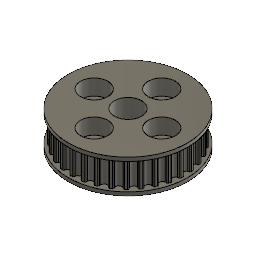
grt_cardan_joint_pulley_33T_20190328 (Autodesk Fusion 360 design; units mm, degrees)
Autodesk Fusion 360 part; units mm, degrees
(part 1 of 2)
sketch "Skizze1" plane through (0, 0, 0) normal (0, 1, 0) x (1, 0, 0)
  line L0 (0, 16.3863) -> (0, 0) construction
  arc A0 (-0.7739, 14.4848) -> (0, 13.9863) centre (0, 14.8363) ccw
  arc A1 (-0.8908, 14.8724) -> (-0.7739, 14.4848) centre (0.61, 15.1135) ccw
  arc A2 (-0.8908, 14.8724) -> (-1.1567, 15.082) centre (-1.1376, 14.8328) ccw
  arc A3 (0, 16.0053) -> (-1.5214, 15.9329) centre (0, 0) ccw construction
  arc A4 (-1.1567, 15.082) -> (-1.4378, 15.0578) centre (0, 0) ccw
  arc A5 (0, 16.3863) -> (-1.5576, 16.3121) centre (0, 0) ccw construction
  line L1 (0, 0) -> (-1.5576, 16.3121) construction
  line L2 (-1.4378, 15.0578) -> (0, 0)
  line L3 (0, 13.9863) -> (0, 0)
  dimension "d2" = 1.14
  dimension "d4" = 0.85
  dimension "d5" = 1.52
  dimension "d6" = 0.25
  dimension "d7" = 0.61
  dimension "d8" = 0.381
  dimension "d12" = 1.26
  dimension "d19" = 5.455
  dimension "d24" = 2.4
  dimension "d131" = 13.9863
  dimension "d133" = 14.6489
  measures "d4" radius of A0
  measures "d5" radius of A1
  measures "d6" radius of A2
  measures "d7" distance of L0
  measures "d19" angle of L0 L1
  measures "d131" distance of L0.end
  measures "d133" distance of L0.end
extrude "Extrusion1" add sketch "Skizze1" along normal blind 7 makes body 1
mirror "Spiegeln1" about plane through (0, 0, -13.9863) normal (1, 0, 0) of bodies 1 makes body 2
combine "Kombinieren1" operation add target body 1 tool bodies 2
pattern_circular "C-Anordnung1" count 33 over 360 about axis through (0, 1.75, 0) along (0, 1, 0) of bodies 1 makes body 3 at (-0.9586, 2.3333, -10.0386) makes body 4 at (-4.2787, 0, -8.8212) makes body 5 at (-5.8708, 0, -7.852) makes body 6 at (-7.2507, 0, -6.5991) makes body 7 at (-8.3685, 0, -5.1076) makes body 8 at (-9.1839, 0, -3.4316) makes body 9 at (-9.6674, 0, -1.6315) makes body 10 at (-9.8014, 0, 0.2276) makes body 11 at (-9.5812, 0, 2.0784) makes body 12 at (-9.0148, 0, 3.8541) makes body 13 at (-8.1225, 0, 5.4905) makes body 14 at (-6.9366, 0, 6.9285) makes body 15 at (-5.5, 0, 8.116) makes body 16 at (-3.8647, 0, 9.0102) makes body 17 at (-2.0896, 0, 9.5788) makes body 18 at (-0.2391, 0, 9.8012) makes body 19 at (1.6201, 0, 9.6693) makes body 20 at (3.4208, 0, 9.1879) makes body 21 at (5.0978, 0, 8.3745) makes body 22 at (6.5906, 0, 7.2584) makes body 23 at (7.8451, 0, 5.88) makes body 24 at (8.8161, 0, 4.289) makes body 25 at (9.4685, 0, 2.543) makes body 26 at (9.7787, 0, 0.7051) makes body 27 at (9.7354, 0, -1.1582) makes body 28 at (9.3403, 0, -2.9797) makes body 29 at (8.6076, 0, -4.6936) makes body 30 at (7.5638, 0, -6.2377) makes body 31 at (6.2466, 0, -7.5565) makes body 32 at (4.7036, 0, -8.6021) makes body 33 at (2.9907, 0, -9.3368) makes body 34 at (0.9586, 2.3333, -10.0386)
combine "Kombinieren2" operation add target body 1 tool bodies 21 20 19 3 18 17 8 15 7 12 9 11 10 16 6 5 14 4 13 31 27 22 23 29 25 24 26 28 30 33 32
sketch "Skizze2" plane through (0, 7, 0) normal (0, 1, 0) x (-1, 0, 0)
  arc A0 (-1.4378, -15.0578) -> (-1.1567, -15.082) centre (0, 0) ccw
  arc A1 (-1.1567, -15.082) -> (-0.8908, -14.8724) centre (-1.1376, -14.8328) ccw
  arc A2 (-0.7739, -14.4848) -> (-0.8908, -14.8724) centre (0.61, -15.1135) ccw
  arc A3 (0.7739, -14.4848) -> (-0.7739, -14.4848) centre (0, -14.8363) ccw
  arc A4 (0.8908, -14.8724) -> (0.7739, -14.4848) centre (-0.61, -15.1135) ccw
  arc A5 (0.8908, -14.8724) -> (1.1567, -15.082) centre (1.1376, -14.8328) ccw
  arc A6 (1.1567, -15.082) -> (1.7185, -15.0284) centre (0, 0) ccw
  arc A7 (1.7185, -15.0284) -> (1.94, -14.7722) centre (1.6901, -14.78) ccw
  arc A8 (1.9814, -14.3695) -> (1.94, -14.7722) centre (3.4592, -14.7249) ccw
  arc A9 (3.5012, -14.0765) -> (1.9814, -14.3695) centre (2.8078, -14.5682) ccw
  arc A10 (3.6893, -14.4351) -> (3.5012, -14.0765) centre (2.2613, -14.9558) ccw
  arc A11 (3.6893, -14.4351) -> (3.9901, -14.5906) centre (3.9242, -14.3494) ccw
  arc A12 (3.9901, -14.5906) -> (4.5316, -14.4316) centre (0, 0) ccw
  arc A13 (4.5316, -14.4316) -> (4.7006, -14.1381) centre (4.4567, -14.1931) ccw
  arc A14 (4.665, -13.7348) -> (4.7006, -14.1381) centre (6.1834, -13.8041) ccw
  arc A15 (6.1019, -13.1596) -> (4.665, -13.7348) centre (5.5141, -13.7736) ccw
  arc A16 (6.3545, -13.476) -> (6.1019, -13.1596) centre (5.0508, -14.2576) ccw
  arc A17 (6.3545, -13.476) -> (6.6793, -13.5718) centre (6.5689, -13.3475) ccw
  arc A18 (6.6793, -13.5718) -> (7.1809, -13.3132) centre (0, 0) ccw
  arc A19 (7.1809, -13.3132) -> (7.2913, -12.9931) centre (7.0622, -13.0932) ccw
  arc A20 (7.18, -12.6037) -> (7.2913, -12.9931) centre (8.6841, -12.3845) ccw
  arc A21 (8.4821, -11.767) -> (7.18, -12.6037) centre (8.0211, -12.4811) ccw
  arc A22 (8.79, -12.0299) -> (8.4821, -11.767) centre (7.6578, -13.044) ccw
  arc A23 (8.79, -12.0299) -> (9.1271, -12.0625) centre (8.9762, -11.8631) ccw
  arc A24 (9.1271, -12.0625) -> (9.5706, -11.7136) centre (0, 0) ccw
  arc A25 (9.5706, -11.7136) -> (9.6185, -11.3784) centre (9.4125, -11.52) ccw
  arc A26 (9.4355, -11.0172) -> (9.6185, -11.3784) centre (10.871, -10.5172) ccw
  arc A27 (10.5557, -9.9491) -> (9.4355, -11.0172) centre (10.2382, -10.7376) ccw
  arc A28 (10.9078, -10.149) -> (10.5557, -9.9491) centre (9.988, -11.3591) ccw
  arc A29 (10.9078, -10.149) -> (11.245, -10.1172) centre (11.0591, -9.95) ccw
  arc A30 (11.245, -10.1172) -> (11.6145, -9.6907) centre (0, 0) ccw
  arc A31 (11.6145, -9.6907) -> (11.598, -9.3524) centre (11.4226, -9.5305) ccw
  arc A32 (11.35, -9.0324) -> (11.598, -9.3524) centre (12.6649, -8.2698) ccw
  arc A33 (12.2478, -7.7716) -> (11.35, -9.0324) centre (12.0853, -8.6059) ccw
  arc A34 (12.6314, -7.9013) -> (12.2478, -7.7716) centre (11.9572, -9.2636) ccw
  arc A35 (12.6314, -7.9013) -> (12.9564, -7.8062) centre (12.7423, -7.6772) ccw
  arc A36 (12.9564, -7.8062) -> (13.2386, -7.3175) centre (0, 0) ccw
  arc A37 (13.2386, -7.3175) -> (13.1584, -6.9885) centre (13.0198, -7.1966) ccw
  arc A38 (12.8543, -6.7211) -> (13.1584, -6.9885) centre (14.0011, -5.7235) ccw
  arc A39 (13.4973, -5.3132) -> (12.8543, -6.7211) centre (13.4956, -6.1632) ccw
  arc A40 (13.8985, -5.368) -> (13.4973, -5.3132) centre (13.4943, -6.8332) ccw
  arc A41 (13.8985, -5.368) -> (14.1996, -5.2131) centre (13.9649, -5.127) ccw
  arc A42 (14.1996, -5.2131) -> (14.3842, -4.6798) centre (0, 0) ccw
  arc A43 (14.3842, -4.6798) -> (14.2432, -4.372) centre (14.1465, -4.6025) ccw
  arc A44 (13.894, -4.167) -> (14.2432, -4.372) centre (14.8313, -2.9703) ccw
  arc A45 (14.2589, -2.6628) -> (13.894, -4.167) centre (14.4181, -3.4978) ccw
  arc A46 (14.6632, -2.6407) -> (14.2589, -2.6628) centre (14.5436, -4.1559) ccw
  arc A47 (14.6632, -2.6407) -> (14.9296, -2.4316) centre (14.6829, -2.3914) ccw
  arc A48 (14.9296, -2.4316) -> (15.0099, -1.873) centre (0, 0) ccw
  arc A49 (15.0099, -1.873) -> (14.8132, -1.5974) centre (14.7618, -1.8421) ccw
  arc A50 (14.4315, -1.4622) -> (14.8132, -1.5974) centre (15.1254, -0.1098) ccw
  arc A51 (14.5052, 0.0838) -> (14.4315, -1.4622) centre (14.8195, -0.7059) ccw
  arc A52 (14.898, 0.1821) -> (14.5052, 0.0838) centre (15.0673, -1.3284) ccw
  arc A53 (14.898, 0.1821) -> (15.12, 0.4378) centre (14.8701, 0.4305) ccw
  arc A54 (15.12, 0.4378) -> (15.0932, 1.0015) centre (0, 0) ccw
  arc A55 (15.0932, 1.0015) -> (14.8478, 1.2349) centre (14.8437, 0.9849) ccw
  arc A56 (14.4475, 1.2954) -> (14.8478, 1.2349) centre (14.8728, 2.7547) ccw
  arc A57 (14.2272, 2.8274) -> (14.4475, 1.2954) centre (14.6853, 2.1114) ccw
  arc A58 (14.5943, 2.9983) -> (14.2272, 2.8274) centre (15.0464, 1.5471) ccw
  arc A59 (14.5943, 2.9983) -> (14.7639, 3.2913) centre (14.5199, 3.2369) ccw
  arc A60 (14.7639, 3.2913) -> (14.6309, 3.8398) centre (0, 0) ccw
  arc A61 (14.6309, 3.8398) -> (14.3458, 4.0225) centre (14.3891, 3.7763) ccw
  arc A62 (13.9412, 4.0062) -> (14.3458, 4.0225) centre (14.0827, 5.5196) ccw
  arc A63 (13.435, 5.4688) -> (13.9412, 4.0062) centre (14.0204, 4.8525) ccw
  arc A64 (13.7631, 5.7061) -> (13.435, 5.4688) centre (14.4818, 4.3667) ccw
  arc A65 (13.7631, 5.7061) -> (13.8742, 6.026) centre (13.6449, 5.9264) ccw
  arc A66 (13.8742, 6.026) -> (13.6398, 6.5393) centre (0, 0) ccw
  arc A67 (13.6398, 6.5393) -> (13.3253, 6.6648) centre (13.4144, 6.4312) ccw
  arc A68 (12.9311, 6.5722) -> (13.3253, 6.6648) centre (12.7836, 8.085) ccw
  arc A69 (12.1572, 7.9126) -> (12.9311, 6.5722) centre (12.8486, 7.4182) ccw
  arc A70 (12.4345, 8.2076) -> (12.1572, 7.9126) centre (13.3936, 7.0285) ccw
  arc A71 (12.4345, 8.2076) -> (12.4831, 8.5428) centre (12.2768, 8.4016) ccw
  arc A72 (12.4831, 8.5428) -> (12.1557, 9.0024) centre (0, 0) ccw
  arc A73 (12.1557, 9.0024) -> (11.8232, 9.0662) centre (11.9548, 8.8537) ccw
  arc A74 (11.4536, 8.9006) -> (11.8232, 9.0662) centre (11.0225, 10.3582) ccw
  arc A75 (10.4401, 10.0704) -> (11.4536, 8.9006) centre (11.2126, 9.7157) ccw
  arc A76 (10.6565, 10.4126) -> (10.4401, 10.0704) centre (11.8215, 9.4362) ccw
  arc A77 (10.6565, 10.4126) -> (10.6408, 10.7508) centre (10.4649, 10.5731) ccw
  arc A78 (10.6408, 10.7508) -> (10.2323, 11.1403) centre (0, 0) ccw
  arc A79 (10.2323, 11.1403) -> (9.8937, 11.1399) centre (10.0632, 10.9561) ccw
  arc A80 (9.5622, 10.9074) -> (9.8937, 11.1399) centre (8.863, 12.2571) ccw
  arc A81 (8.3456, 11.8642) -> (9.5622, 10.9074) centre (9.1712, 11.6622) ccw
  arc A82 (8.4933, 12.2412) -> (8.3456, 11.8642) centre (9.822, 11.5029) ccw
  arc A83 (8.4933, 12.2412) -> (8.4139, 12.5703) centre (8.2748, 12.3626) ccw
  arc A84 (8.4139, 12.5703) -> (7.9391, 12.8754) centre (0, 0) ccw
  arc A85 (7.9391, 12.8754) -> (7.6067, 12.811) centre (7.8079, 12.6626) ccw
  arc A86 (7.3252, 12.52) -> (7.6067, 12.811) centre (6.3832, 13.7129) ccw
  arc A87 (5.9494, 13.2292) -> (7.3252, 12.52) centre (6.7984, 13.1871) ccw
  arc A88 (6.0232, 13.6273) -> (5.9494, 13.2292) centre (7.4676, 13.1539) ccw
  arc A89 (6.0232, 13.6273) -> (5.8829, 13.9355) centre (5.7856, 13.7052) ccw
  arc A90 (5.8829, 13.9355) -> (5.359, 14.1452) centre (0, 0) ccw
  arc A91 (5.359, 14.1452) -> (5.0447, 14.019) centre (5.2704, 13.9114) ccw
  arc A92 (4.8234, 13.68) -> (5.0447, 14.019) centre (3.6727, 14.6731) ccw
  arc A93 (3.3383, 14.1161) -> (4.8234, 13.68) centre (4.1799, 14.2354) ccw
  arc A94 (3.3354, 14.5209) -> (3.3383, 14.1161) centre (4.8432, 14.3294) ccw
  arc A95 (3.3354, 14.5209) -> (3.1392, 14.797) centre (3.0874, 14.5524) ccw
  arc A96 (3.1392, 14.797) -> (2.5851, 14.9038) centre (0, 0) ccw
  arc A97 (2.5851, 14.9038) -> (2.3004, 14.7204) centre (2.5424, 14.6575) ccw
  arc A98 (2.1472, 14.3456) -> (2.3004, 14.7204) centre (0.8294, 15.103) ccw
  arc A99 (0.6065, 14.4927) -> (2.1472, 14.3456) centre (1.4103, 14.7692) ccw
  arc A100 (0.527, 14.8898) -> (0.6065, 14.4927) centre (2.0439, 14.987) ccw
  arc A101 (0.527, 14.8898) -> (0.2822, 15.1237) centre (0.2775, 14.8738) ccw
  arc A102 (0.2822, 15.1237) -> (-0.2822, 15.1237) centre (0, 0) ccw
  arc A103 (-0.2822, 15.1237) -> (-0.527, 14.8898) centre (-0.2775, 14.8738) ccw
  arc A104 (-0.6065, 14.4927) -> (-0.527, 14.8898) centre (-2.0439, 14.987) ccw
  arc A105 (-2.1472, 14.3456) -> (-0.6065, 14.4927) centre (-1.4103, 14.7692) ccw
  arc A106 (-2.3004, 14.7204) -> (-2.1472, 14.3456) centre (-0.8294, 15.103) ccw
  arc A107 (-2.3004, 14.7204) -> (-2.5851, 14.9038) centre (-2.5424, 14.6575) ccw
  arc A108 (-2.5851, 14.9038) -> (-3.1392, 14.797) centre (0, 0) ccw
  arc A109 (-3.1392, 14.797) -> (-3.3354, 14.5209) centre (-3.0874, 14.5524) ccw
  arc A110 (-3.3383, 14.1161) -> (-3.3354, 14.5209) centre (-4.8432, 14.3294) ccw
  arc A111 (-4.8234, 13.68) -> (-3.3383, 14.1161) centre (-4.1799, 14.2354) ccw
  arc A112 (-5.0447, 14.019) -> (-4.8234, 13.68) centre (-3.6727, 14.6731) ccw
  arc A113 (-5.0447, 14.019) -> (-5.359, 14.1452) centre (-5.2704, 13.9114) ccw
  arc A114 (-5.359, 14.1452) -> (-5.8829, 13.9355) centre (0, 0) ccw
  arc A115 (-5.8829, 13.9355) -> (-6.0232, 13.6273) centre (-5.7856, 13.7052) ccw
  arc A116 (-5.9494, 13.2292) -> (-6.0232, 13.6273) centre (-7.4676, 13.1539) ccw
  arc A117 (-7.3252, 12.52) -> (-5.9494, 13.2292) centre (-6.7984, 13.1871) ccw
  arc A118 (-7.6067, 12.811) -> (-7.3252, 12.52) centre (-6.3832, 13.7129) ccw
  arc A119 (-7.6067, 12.811) -> (-7.9391, 12.8754) centre (-7.8079, 12.6626) ccw
  arc A120 (-7.9391, 12.8754) -> (-8.4139, 12.5703) centre (0, 0) ccw
  arc A121 (-8.4139, 12.5703) -> (-8.4933, 12.2412) centre (-8.2748, 12.3626) ccw
  arc A122 (-8.3456, 11.8642) -> (-8.4933, 12.2412) centre (-9.822, 11.5029) ccw
  arc A123 (-9.5622, 10.9074) -> (-8.3456, 11.8642) centre (-9.1712, 11.6622) ccw
  arc A124 (-9.8937, 11.1399) -> (-9.5622, 10.9074) centre (-8.863, 12.2571) ccw
  arc A125 (-9.8937, 11.1399) -> (-10.2323, 11.1403) centre (-10.0632, 10.9561) ccw
  arc A126 (-10.2323, 11.1403) -> (-10.6408, 10.7508) centre (0, 0) ccw
  arc A127 (-10.6408, 10.7508) -> (-10.6565, 10.4126) centre (-10.4649, 10.5731) ccw
  arc A128 (-10.4401, 10.0704) -> (-10.6565, 10.4126) centre (-11.8215, 9.4362) ccw
  arc A129 (-11.4536, 8.9006) -> (-10.4401, 10.0704) centre (-11.2126, 9.7157) ccw
  arc A130 (-11.8232, 9.0662) -> (-11.4536, 8.9006) centre (-11.0225, 10.3582) ccw
  arc A131 (-11.8232, 9.0662) -> (-12.1557, 9.0024) centre (-11.9548, 8.8537) ccw
  arc A132 (-12.1557, 9.0024) -> (-12.4831, 8.5428) centre (0, 0) ccw
  arc A133 (-12.4831, 8.5428) -> (-12.4345, 8.2076) centre (-12.2768, 8.4016) ccw
  arc A134 (-12.1572, 7.9126) -> (-12.4345, 8.2076) centre (-13.3936, 7.0285) ccw
  arc A135 (-12.9311, 6.5722) -> (-12.1572, 7.9126) centre (-12.8486, 7.4182) ccw
  arc A136 (-13.3253, 6.6648) -> (-12.9311, 6.5722) centre (-12.7836, 8.085) ccw
  arc A137 (-13.3253, 6.6648) -> (-13.6398, 6.5393) centre (-13.4144, 6.4312) ccw
  arc A138 (-13.6398, 6.5393) -> (-13.8742, 6.026) centre (0, 0) ccw
  arc A139 (-13.8742, 6.026) -> (-13.7631, 5.7061) centre (-13.6449, 5.9264) ccw
  arc A140 (-13.435, 5.4688) -> (-13.7631, 5.7061) centre (-14.4818, 4.3667) ccw
  arc A141 (-13.9412, 4.0062) -> (-13.435, 5.4688) centre (-14.0204, 4.8525) ccw
  arc A142 (-14.3458, 4.0225) -> (-13.9412, 4.0062) centre (-14.0827, 5.5196) ccw
  arc A143 (-14.3458, 4.0225) -> (-14.6309, 3.8398) centre (-14.3891, 3.7763) ccw
  arc A144 (-14.6309, 3.8398) -> (-14.7639, 3.2913) centre (0, 0) ccw
  arc A145 (-14.7639, 3.2913) -> (-14.5943, 2.9983) centre (-14.5199, 3.2369) ccw
  arc A146 (-14.2272, 2.8274) -> (-14.5943, 2.9983) centre (-15.0464, 1.5471) ccw
  arc A147 (-14.4475, 1.2954) -> (-14.2272, 2.8274) centre (-14.6853, 2.1114) ccw
  arc A148 (-14.8478, 1.2349) -> (-14.4475, 1.2954) centre (-14.8728, 2.7547) ccw
  arc A149 (-14.8478, 1.2349) -> (-15.0932, 1.0015) centre (-14.8437, 0.9849) ccw
  arc A150 (-15.0932, 1.0015) -> (-15.12, 0.4378) centre (0, 0) ccw
  arc A151 (-15.12, 0.4378) -> (-14.898, 0.1821) centre (-14.8701, 0.4305) ccw
  arc A152 (-14.5052, 0.0838) -> (-14.898, 0.1821) centre (-15.0673, -1.3284) ccw
  arc A153 (-14.4315, -1.4622) -> (-14.5052, 0.0838) centre (-14.8195, -0.7059) ccw
  arc A154 (-14.8132, -1.5974) -> (-14.4315, -1.4622) centre (-15.1254, -0.1098) ccw
  arc A155 (-14.8132, -1.5974) -> (-15.0099, -1.873) centre (-14.7618, -1.8421) ccw
  arc A156 (-15.0099, -1.873) -> (-14.9296, -2.4316) centre (0, 0) ccw
  arc A157 (-14.9296, -2.4316) -> (-14.6632, -2.6407) centre (-14.6829, -2.3914) ccw
  arc A158 (-14.2589, -2.6628) -> (-14.6632, -2.6407) centre (-14.5436, -4.1559) ccw
  arc A159 (-13.894, -4.167) -> (-14.2589, -2.6628) centre (-14.4181, -3.4978) ccw
  arc A160 (-14.2432, -4.372) -> (-13.894, -4.167) centre (-14.8313, -2.9703) ccw
  arc A161 (-14.2432, -4.372) -> (-14.3842, -4.6798) centre (-14.1465, -4.6025) ccw
  arc A162 (-14.3842, -4.6798) -> (-14.1996, -5.2131) centre (0, 0) ccw
  arc A163 (-14.1996, -5.2131) -> (-13.8985, -5.368) centre (-13.9649, -5.127) ccw
  arc A164 (-13.4973, -5.3132) -> (-13.8985, -5.368) centre (-13.4943, -6.8332) ccw
  arc A165 (-12.8543, -6.7211) -> (-13.4973, -5.3132) centre (-13.4956, -6.1632) ccw
  arc A166 (-13.1584, -6.9885) -> (-12.8543, -6.7211) centre (-14.0011, -5.7235) ccw
  arc A167 (-13.1584, -6.9885) -> (-13.2386, -7.3175) centre (-13.0198, -7.1966) ccw
  arc A168 (-13.2386, -7.3175) -> (-12.9564, -7.8062) centre (0, 0) ccw
  arc A169 (-12.9564, -7.8062) -> (-12.6314, -7.9013) centre (-12.7423, -7.6772) ccw
  arc A170 (-12.2478, -7.7716) -> (-12.6314, -7.9013) centre (-11.9572, -9.2636) ccw
  arc A171 (-11.35, -9.0324) -> (-12.2478, -7.7716) centre (-12.0853, -8.6059) ccw
  arc A172 (-11.598, -9.3524) -> (-11.35, -9.0324) centre (-12.6649, -8.2698) ccw
  arc A173 (-11.598, -9.3524) -> (-11.6145, -9.6907) centre (-11.4226, -9.5305) ccw
  arc A174 (-11.6145, -9.6907) -> (-11.245, -10.1172) centre (0, 0) ccw
  arc A175 (-11.245, -10.1172) -> (-10.9078, -10.149) centre (-11.0591, -9.95) ccw
  arc A176 (-10.5557, -9.9491) -> (-10.9078, -10.149) centre (-9.988, -11.3591) ccw
  arc A177 (-9.4355, -11.0172) -> (-10.5557, -9.9491) centre (-10.2382, -10.7376) ccw
  arc A178 (-9.6185, -11.3784) -> (-9.4355, -11.0172) centre (-10.871, -10.5172) ccw
  arc A179 (-9.6185, -11.3784) -> (-9.5706, -11.7136) centre (-9.4125, -11.52) ccw
  circle A180 centre (0, 0) radius 16.3753
  arc A181 (-9.5706, -11.7136) -> (-9.1271, -12.0625) centre (0, 0) ccw
  arc A182 (-9.1271, -12.0625) -> (-8.79, -12.0299) centre (-8.9762, -11.8631) ccw
  arc A183 (-8.4821, -11.767) -> (-8.79, -12.0299) centre (-7.6578, -13.044) ccw
  arc A184 (-7.18, -12.6037) -> (-8.4821, -11.767) centre (-8.0211, -12.4811) ccw
  arc A185 (-7.2913, -12.9931) -> (-7.18, -12.6037) centre (-8.6841, -12.3845) ccw
  arc A186 (-7.2913, -12.9931) -> (-7.1809, -13.3132) centre (-7.0622, -13.0932) ccw
  arc A187 (-7.1809, -13.3132) -> (-6.6793, -13.5718) centre (0, 0) ccw
  arc A188 (-6.6793, -13.5718) -> (-6.3545, -13.476) centre (-6.5689, -13.3475) ccw
  arc A189 (-6.1019, -13.1596) -> (-6.3545, -13.476) centre (-5.0508, -14.2576) ccw
  arc A190 (-4.665, -13.7348) -> (-6.1019, -13.1596) centre (-5.5141, -13.7736) ccw
  arc A191 (-4.7006, -14.1381) -> (-4.665, -13.7348) centre (-6.1834, -13.8041) ccw
  arc A192 (-4.7006, -14.1381) -> (-4.5316, -14.4316) centre (-4.4567, -14.1931) ccw
  arc A193 (-4.5316, -14.4316) -> (-4.2616, -14.5136) centre (0, 0) ccw
  line L0 (-4.2616, -14.5136) -> (0, 0)
  line L1 (0, 0) -> (-1.4378, -15.0578)
  dimension "d30" = 32.7507
  measures "d30" diameter of A180
extrude "Extrusion2" add sketch "Skizze2" along normal blind 1 contours A0 A1 A2 A3 A4 A5 A6 A7 A8 A9 A10 A11 A12 A13 A14 A15 A16 A17 A18 A19 A20 A21 A22 A23 A24 A25 A26 A27 A28 A29 A30 A31 A32 A33 A34 A35 A36 A37 A38 A39 A40 A41 A42 A43 A44 A45 A46 A47 A48 A49 A50 A51 A52 A53 A54 A55 A56 A57 A58 A59 A60 A61 A62 A63 A64 A65 A66 A67 A68 A69 A70 A71 A72 A73 A74 A75 A76 A77 A78 A79 A80 A81 A82 A83 A84 A85 A86 A87 A88 A89 A90 A91 A92 A93 A94 A95 A96 A97 A98 A99 A100 A101 A102 A103 A104 A105 A106 A107 A108 A109 A110 A111 A112 A113 A114 A115 A116 A117 A118 A119 A120 A121 A122 A123 A124 A125 A126 A127 A128 A129 A130 A131 A132 A133 A134 A135 A136 A137 A138 A139 A140 A141 A142 A143 A144 A145 A146 A147 A148 A149 A150 A151 A152 A153 A154 A155 A156 A157 A158 A159 A160 A161 A162 A163 A164 A165 A166 A167 A168 A169 A170 A171 A172 A173 A174 A175 A176 A177 A178 A179 A181 A182 A183 A184 A185 A186 A187 A188 A189 A190 A191 A192 A193 L0 L1 | A180 bodies 1 34
sketch "Skizze3" plane through (0, 0, 0) normal (0, -1, 0) x (1, 0, 0)
  arc A0 (9.5706, -11.7136) -> (9.6185, -11.3784) centre (9.4125, -11.52) ccw
  arc A1 (9.4355, -11.0172) -> (9.6185, -11.3784) centre (10.871, -10.5172) ccw
  arc A2 (10.5557, -9.9491) -> (9.4355, -11.0172) centre (10.2382, -10.7376) ccw
  arc A3 (10.9078, -10.149) -> (10.5557, -9.9491) centre (9.988, -11.3591) ccw
  arc A4 (10.9078, -10.149) -> (11.245, -10.1172) centre (11.0591, -9.95) ccw
  arc A5 (11.245, -10.1172) -> (11.6145, -9.6907) centre (0, 0) ccw
  arc A6 (11.6145, -9.6907) -> (11.598, -9.3524) centre (11.4226, -9.5305) ccw
  arc A7 (11.35, -9.0324) -> (11.598, -9.3524) centre (12.6649, -8.2698) ccw
  arc A8 (12.2478, -7.7716) -> (11.35, -9.0324) centre (12.0853, -8.6059) ccw
  arc A9 (12.6314, -7.9013) -> (12.2478, -7.7716) centre (11.9572, -9.2636) ccw
  arc A10 (12.6314, -7.9013) -> (12.9564, -7.8062) centre (12.7423, -7.6772) ccw
  arc A11 (12.9564, -7.8062) -> (13.2386, -7.3175) centre (0, 0) ccw
  arc A12 (13.2386, -7.3175) -> (13.1584, -6.9885) centre (13.0198, -7.1966) ccw
  arc A13 (12.8543, -6.7211) -> (13.1584, -6.9885) centre (14.0011, -5.7235) ccw
  arc A14 (13.4973, -5.3132) -> (12.8543, -6.7211) centre (13.4956, -6.1632) ccw
  arc A15 (13.8985, -5.368) -> (13.4973, -5.3132) centre (13.4943, -6.8332) ccw
  arc A16 (13.8985, -5.368) -> (14.1996, -5.2131) centre (13.9649, -5.127) ccw
  arc A17 (14.1996, -5.2131) -> (14.3842, -4.6798) centre (0, 0) ccw
  arc A18 (14.3842, -4.6798) -> (14.2432, -4.372) centre (14.1465, -4.6025) ccw
  arc A19 (13.894, -4.167) -> (14.2432, -4.372) centre (14.8313, -2.9703) ccw
  arc A20 (14.2589, -2.6628) -> (13.894, -4.167) centre (14.4181, -3.4978) ccw
  arc A21 (14.6632, -2.6407) -> (14.2589, -2.6628) centre (14.5436, -4.1559) ccw
  arc A22 (14.6632, -2.6407) -> (14.9296, -2.4316) centre (14.6829, -2.3914) ccw
  arc A23 (14.9296, -2.4316) -> (15.0099, -1.873) centre (0, 0) ccw
  arc A24 (15.0099, -1.873) -> (14.8132, -1.5974) centre (14.7618, -1.8421) ccw
  arc A25 (14.4315, -1.4622) -> (14.8132, -1.5974) centre (15.1254, -0.1098) ccw
  arc A26 (14.5052, 0.0838) -> (14.4315, -1.4622) centre (14.8195, -0.7059) ccw
  arc A27 (14.898, 0.1821) -> (14.5052, 0.0838) centre (15.0673, -1.3284) ccw
  arc A28 (14.898, 0.1821) -> (15.12, 0.4378) centre (14.8701, 0.4305) ccw
  arc A29 (15.12, 0.4378) -> (15.0932, 1.0015) centre (0, 0) ccw
  arc A30 (15.0932, 1.0015) -> (14.8478, 1.2349) centre (14.8437, 0.9849) ccw
  arc A31 (14.4475, 1.2954) -> (14.8478, 1.2349) centre (14.8728, 2.7547) ccw
  arc A32 (14.2272, 2.8274) -> (14.4475, 1.2954) centre (14.6853, 2.1114) ccw
  arc A33 (14.5943, 2.9983) -> (14.2272, 2.8274) centre (15.0464, 1.5471) ccw
  arc A34 (14.5943, 2.9983) -> (14.7639, 3.2913) centre (14.5199, 3.2369) ccw
  arc A35 (14.7639, 3.2913) -> (14.6309, 3.8398) centre (0, 0) ccw
  arc A36 (14.6309, 3.8398) -> (14.3458, 4.0225) centre (14.3891, 3.7763) ccw
  arc A37 (13.9412, 4.0062) -> (14.3458, 4.0225) centre (14.0827, 5.5196) ccw
  arc A38 (13.435, 5.4688) -> (13.9412, 4.0062) centre (14.0204, 4.8525) ccw
  arc A39 (13.7631, 5.7061) -> (13.435, 5.4688) centre (14.4818, 4.3667) ccw
  arc A40 (13.7631, 5.7061) -> (13.8742, 6.026) centre (13.6449, 5.9264) ccw
  arc A41 (13.8742, 6.026) -> (13.6398, 6.5393) centre (0, 0) ccw
  arc A42 (13.6398, 6.5393) -> (13.3253, 6.6648) centre (13.4144, 6.4312) ccw
  arc A43 (12.9311, 6.5722) -> (13.3253, 6.6648) centre (12.7836, 8.085) ccw
  arc A44 (12.1572, 7.9126) -> (12.9311, 6.5722) centre (12.8486, 7.4182) ccw
  arc A45 (12.4345, 8.2076) -> (12.1572, 7.9126) centre (13.3936, 7.0285) ccw
  arc A46 (12.4345, 8.2076) -> (12.4831, 8.5428) centre (12.2768, 8.4016) ccw
  arc A47 (12.4831, 8.5428) -> (12.1557, 9.0024) centre (0, 0) ccw
  arc A48 (12.1557, 9.0024) -> (11.8232, 9.0662) centre (11.9548, 8.8537) ccw
  arc A49 (11.4536, 8.9006) -> (11.8232, 9.0662) centre (11.0225, 10.3582) ccw
  arc A50 (10.4401, 10.0704) -> (11.4536, 8.9006) centre (11.2126, 9.7157) ccw
  arc A51 (10.6565, 10.4126) -> (10.4401, 10.0704) centre (11.8215, 9.4362) ccw
  arc A52 (10.6565, 10.4126) -> (10.6408, 10.7508) centre (10.4649, 10.5731) ccw
  arc A53 (10.6408, 10.7508) -> (10.2323, 11.1403) centre (0, 0) ccw
  arc A54 (10.2323, 11.1403) -> (9.8937, 11.1399) centre (10.0632, 10.9561) ccw
  arc A55 (9.5622, 10.9074) -> (9.8937, 11.1399) centre (8.863, 12.2571) ccw
  arc A56 (8.3456, 11.8642) -> (9.5622, 10.9074) centre (9.1712, 11.6622) ccw
  arc A57 (8.4933, 12.2412) -> (8.3456, 11.8642) centre (9.822, 11.5029) ccw
  arc A58 (8.4933, 12.2412) -> (8.4139, 12.5703) centre (8.2748, 12.3626) ccw
  arc A59 (8.4139, 12.5703) -> (7.9391, 12.8754) centre (0, 0) ccw
  arc A60 (7.9391, 12.8754) -> (7.6067, 12.811) centre (7.8079, 12.6626) ccw
  arc A61 (7.3252, 12.52) -> (7.6067, 12.811) centre (6.3832, 13.7129) ccw
  arc A62 (5.9494, 13.2292) -> (7.3252, 12.52) centre (6.7984, 13.1871) ccw
  arc A63 (6.0232, 13.6273) -> (5.9494, 13.2292) centre (7.4676, 13.1539) ccw
  arc A64 (6.0232, 13.6273) -> (5.8829, 13.9355) centre (5.7856, 13.7052) ccw
  arc A65 (5.8829, 13.9355) -> (5.359, 14.1452) centre (0, 0) ccw
  arc A66 (5.359, 14.1452) -> (5.0447, 14.019) centre (5.2704, 13.9114) ccw
  arc A67 (4.8234, 13.68) -> (5.0447, 14.019) centre (3.6727, 14.6731) ccw
  arc A68 (3.3383, 14.1161) -> (4.8234, 13.68) centre (4.1799, 14.2354) ccw
  arc A69 (3.3354, 14.5209) -> (3.3383, 14.1161) centre (4.8432, 14.3294) ccw
  arc A70 (3.3354, 14.5209) -> (3.1392, 14.797) centre (3.0874, 14.5524) ccw
  arc A71 (3.1392, 14.797) -> (2.5851, 14.9038) centre (0, 0) ccw
  arc A72 (2.5851, 14.9038) -> (2.3004, 14.7204) centre (2.5424, 14.6575) ccw
  arc A73 (2.1472, 14.3456) -> (2.3004, 14.7204) centre (0.8294, 15.103) ccw
  arc A74 (0.6065, 14.4927) -> (2.1472, 14.3456) centre (1.4103, 14.7692) ccw
  arc A75 (0.527, 14.8898) -> (0.6065, 14.4927) centre (2.0439, 14.987) ccw
  arc A76 (0.527, 14.8898) -> (0.2822, 15.1237) centre (0.2775, 14.8738) ccw
  arc A77 (0.2822, 15.1237) -> (-0.2822, 15.1237) centre (0, 0) ccw
  arc A78 (-0.2822, 15.1237) -> (-0.527, 14.8898) centre (-0.2775, 14.8738) ccw
  arc A79 (-0.6065, 14.4927) -> (-0.527, 14.8898) centre (-2.0439, 14.987) ccw
  arc A80 (-2.1472, 14.3456) -> (-0.6065, 14.4927) centre (-1.4103, 14.7692) ccw
  arc A81 (-2.3004, 14.7204) -> (-2.1472, 14.3456) centre (-0.8294, 15.103) ccw
  arc A82 (-2.3004, 14.7204) -> (-2.5851, 14.9038) centre (-2.5424, 14.6575) ccw
  arc A83 (-2.5851, 14.9038) -> (-3.1392, 14.797) centre (0, 0) ccw
  arc A84 (-3.1392, 14.797) -> (-3.3354, 14.5209) centre (-3.0874, 14.5524) ccw
  arc A85 (-3.3383, 14.1161) -> (-3.3354, 14.5209) centre (-4.8432, 14.3294) ccw
  arc A86 (-4.8234, 13.68) -> (-3.3383, 14.1161) centre (-4.1799, 14.2354) ccw
  arc A87 (-5.0447, 14.019) -> (-4.8234, 13.68) centre (-3.6727, 14.6731) ccw
  arc A88 (-5.0447, 14.019) -> (-5.359, 14.1452) centre (-5.2704, 13.9114) ccw
  arc A89 (-5.359, 14.1452) -> (-5.8829, 13.9355) centre (0, 0) ccw
  arc A90 (-5.8829, 13.9355) -> (-6.0232, 13.6273) centre (-5.7856, 13.7052) ccw
  arc A91 (-5.9494, 13.2292) -> (-6.0232, 13.6273) centre (-7.4676, 13.1539) ccw
  arc A92 (-7.3252, 12.52) -> (-5.9494, 13.2292) centre (-6.7984, 13.1871) ccw
  arc A93 (-7.6067, 12.811) -> (-7.3252, 12.52) centre (-6.3832, 13.7129) ccw
  arc A94 (-7.6067, 12.811) -> (-7.9391, 12.8754) centre (-7.8079, 12.6626) ccw
  arc A95 (-7.9391, 12.8754) -> (-8.4139, 12.5703) centre (0, 0) ccw
  arc A96 (-8.4139, 12.5703) -> (-8.4933, 12.2412) centre (-8.2748, 12.3626) ccw
  arc A97 (-8.3456, 11.8642) -> (-8.4933, 12.2412) centre (-9.822, 11.5029) ccw
  arc A98 (-9.5622, 10.9074) -> (-8.3456, 11.8642) centre (-9.1712, 11.6622) ccw
  arc A99 (-9.8937, 11.1399) -> (-9.5622, 10.9074) centre (-8.863, 12.2571) ccw
  arc A100 (-9.8937, 11.1399) -> (-10.2323, 11.1403) centre (-10.0632, 10.9561) ccw
  arc A101 (-10.2323, 11.1403) -> (-10.6408, 10.7508) centre (0, 0) ccw
  arc A102 (-10.6408, 10.7508) -> (-10.6565, 10.4126) centre (-10.4649, 10.5731) ccw
  arc A103 (-10.4401, 10.0704) -> (-10.6565, 10.4126) centre (-11.8215, 9.4362) ccw
  arc A104 (-11.4536, 8.9006) -> (-10.4401, 10.0704) centre (-11.2126, 9.7157) ccw
  arc A105 (-11.8232, 9.0662) -> (-11.4536, 8.9006) centre (-11.0225, 10.3582) ccw
  arc A106 (-11.8232, 9.0662) -> (-12.1557, 9.0024) centre (-11.9548, 8.8537) ccw
  arc A107 (-12.1557, 9.0024) -> (-12.4831, 8.5428) centre (0, 0) ccw
  arc A108 (-12.4831, 8.5428) -> (-12.4345, 8.2076) centre (-12.2768, 8.4016) ccw
  arc A109 (-12.1572, 7.9126) -> (-12.4345, 8.2076) centre (-13.3936, 7.0285) ccw
  arc A110 (-12.9311, 6.5722) -> (-12.1572, 7.9126) centre (-12.8486, 7.4182) ccw
  arc A111 (-13.3253, 6.6648) -> (-12.9311, 6.5722) centre (-12.7836, 8.085) ccw
  arc A112 (-13.3253, 6.6648) -> (-13.6398, 6.5393) centre (-13.4144, 6.4312) ccw
  arc A113 (-13.6398, 6.5393) -> (-13.8742, 6.026) centre (0, 0) ccw
  arc A114 (-13.8742, 6.026) -> (-13.7631, 5.7061) centre (-13.6449, 5.9264) ccw
  arc A115 (-13.435, 5.4688) -> (-13.7631, 5.7061) centre (-14.4818, 4.3667) ccw
  arc A116 (-13.9412, 4.0062) -> (-13.435, 5.4688) centre (-14.0204, 4.8525) ccw
  arc A117 (-14.3458, 4.0225) -> (-13.9412, 4.0062) centre (-14.0827, 5.5196) ccw
  arc A118 (-14.3458, 4.0225) -> (-14.6309, 3.8398) centre (-14.3891, 3.7763) ccw
  arc A119 (-14.6309, 3.8398) -> (-14.7639, 3.2913) centre (0, 0) ccw
  arc A120 (-14.7639, 3.2913) -> (-14.5943, 2.9983) centre (-14.5199, 3.2369) ccw
  arc A121 (-14.2272, 2.8274) -> (-14.5943, 2.9983) centre (-15.0464, 1.5471) ccw
  arc A122 (-14.4475, 1.2954) -> (-14.2272, 2.8274) centre (-14.6853, 2.1114) ccw
  arc A123 (-14.8478, 1.2349) -> (-14.4475, 1.2954) centre (-14.8728, 2.7547) ccw
  arc A124 (-14.8478, 1.2349) -> (-15.0932, 1.0015) centre (-14.8437, 0.9849) ccw
  arc A125 (-15.0932, 1.0015) -> (-15.12, 0.4378) centre (0, 0) ccw
  arc A126 (-15.12, 0.4378) -> (-14.898, 0.1821) centre (-14.8701, 0.4305) ccw
  arc A127 (-14.5052, 0.0838) -> (-14.898, 0.1821) centre (-15.0673, -1.3284) ccw
  arc A128 (-14.4315, -1.4622) -> (-14.5052, 0.0838) centre (-14.8195, -0.7059) ccw
  arc A129 (-14.8132, -1.5974) -> (-14.4315, -1.4622) centre (-15.1254, -0.1098) ccw
  arc A130 (-14.8132, -1.5974) -> (-15.0099, -1.873) centre (-14.7618, -1.8421) ccw
  arc A131 (-15.0099, -1.873) -> (-14.9296, -2.4316) centre (0, 0) ccw
  arc A132 (-14.9296, -2.4316) -> (-14.6632, -2.6407) centre (-14.6829, -2.3914) ccw
  arc A133 (-14.2589, -2.6628) -> (-14.6632, -2.6407) centre (-14.5436, -4.1559) ccw
  arc A134 (-13.894, -4.167) -> (-14.2589, -2.6628) centre (-14.4181, -3.4978) ccw
  arc A135 (-14.2432, -4.372) -> (-13.894, -4.167) centre (-14.8313, -2.9703) ccw
  arc A136 (-14.2432, -4.372) -> (-14.3842, -4.6798) centre (-14.1465, -4.6025) ccw
  arc A137 (-14.3842, -4.6798) -> (-14.1996, -5.2131) centre (0, 0) ccw
  arc A138 (-14.1996, -5.2131) -> (-13.8985, -5.368) centre (-13.9649, -5.127) ccw
  arc A139 (-13.4973, -5.3132) -> (-13.8985, -5.368) centre (-13.4943, -6.8332) ccw
  arc A140 (-12.8543, -6.7211) -> (-13.4973, -5.3132) centre (-13.4956, -6.1632) ccw
  arc A141 (-13.1584, -6.9885) -> (-12.8543, -6.7211) centre (-14.0011, -5.7235) ccw
  arc A142 (-13.1584, -6.9885) -> (-13.2386, -7.3175) centre (-13.0198, -7.1966) ccw
  arc A143 (-13.2386, -7.3175) -> (-12.9564, -7.8062) centre (0, 0) ccw
  arc A144 (-12.9564, -7.8062) -> (-12.6314, -7.9013) centre (-12.7423, -7.6772) ccw
  arc A145 (-12.2478, -7.7716) -> (-12.6314, -7.9013) centre (-11.9572, -9.2636) ccw
  arc A146 (-11.35, -9.0324) -> (-12.2478, -7.7716) centre (-12.0853, -8.6059) ccw
  arc A147 (-11.598, -9.3524) -> (-11.35, -9.0324) centre (-12.6649, -8.2698) ccw
  arc A148 (-11.598, -9.3524) -> (-11.6145, -9.6907) centre (-11.4226, -9.5305) ccw
  arc A149 (-11.6145, -9.6907) -> (-11.245, -10.1172) centre (0, 0) ccw
  arc A150 (-11.245, -10.1172) -> (-10.9078, -10.149) centre (-11.0591, -9.95) ccw
  arc A151 (-10.5557, -9.9491) -> (-10.9078, -10.149) centre (-9.988, -11.3591) ccw
  arc A152 (-9.4355, -11.0172) -> (-10.5557, -9.9491) centre (-10.2382, -10.7376) ccw
  arc A153 (-9.6185, -11.3784) -> (-9.4355, -11.0172) centre (-10.871, -10.5172) ccw
  arc A154 (-9.6185, -11.3784) -> (-9.5706, -11.7136) centre (-9.4125, -11.52) ccw
  arc A155 (-9.5706, -11.7136) -> (-9.1271, -12.0625) centre (0, 0) ccw
  arc A156 (-9.1271, -12.0625) -> (-8.79, -12.0299) centre (-8.9762, -11.8631) ccw
  arc A157 (-8.4821, -11.767) -> (-8.79, -12.0299) centre (-7.6578, -13.044) ccw
  arc A158 (-7.18, -12.6037) -> (-8.4821, -11.767) centre (-8.0211, -12.4811) ccw
  arc A159 (-7.2913, -12.9931) -> (-7.18, -12.6037) centre (-8.6841, -12.3845) ccw
  arc A160 (-7.2913, -12.9931) -> (-7.1809, -13.3132) centre (-7.0622, -13.0932) ccw
  arc A161 (-7.1809, -13.3132) -> (-6.6793, -13.5718) centre (0, 0) ccw
  arc A162 (-6.6793, -13.5718) -> (-6.3545, -13.476) centre (-6.5689, -13.3475) ccw
  arc A163 (-6.1019, -13.1596) -> (-6.3545, -13.476) centre (-5.0508, -14.2576) ccw
  arc A164 (-4.665, -13.7348) -> (-6.1019, -13.1596) centre (-5.5141, -13.7736) ccw
  arc A165 (-4.7006, -14.1381) -> (-4.665, -13.7348) centre (-6.1834, -13.8041) ccw
  arc A166 (-4.7006, -14.1381) -> (-4.5316, -14.4316) centre (-4.4567, -14.1931) ccw
  arc A167 (-4.5316, -14.4316) -> (-3.9901, -14.5906) centre (0, 0) ccw
  arc A168 (-3.9901, -14.5906) -> (-3.6893, -14.4351) centre (-3.9242, -14.3494) ccw
  arc A169 (-3.5012, -14.0765) -> (-3.6893, -14.4351) centre (-2.2613, -14.9558) ccw
  arc A170 (-1.9814, -14.3695) -> (-3.5012, -14.0765) centre (-2.8078, -14.5682) ccw
  arc A171 (-1.94, -14.7722) -> (-1.9814, -14.3695) centre (-3.4592, -14.7249) ccw
  arc A172 (-1.94, -14.7722) -> (-1.7185, -15.0284) centre (-1.6901, -14.78) ccw
  arc A173 (-1.7185, -15.0284) -> (-1.1567, -15.082) centre (0, 0) ccw
  arc A174 (-1.1567, -15.082) -> (-0.8908, -14.8724) centre (-1.1376, -14.8328) ccw
  arc A175 (-0.7739, -14.4848) -> (-0.8908, -14.8724) centre (0.61, -15.1135) ccw
  arc A176 (0.7739, -14.4848) -> (-0.7739, -14.4848) centre (0, -14.8363) ccw
  arc A177 (0.8908, -14.8724) -> (0.7739, -14.4848) centre (-0.61, -15.1135) ccw
  arc A178 (0.8908, -14.8724) -> (1.1567, -15.082) centre (1.1376, -14.8328) ccw
  arc A179 (1.1567, -15.082) -> (1.7185, -15.0284) centre (0, 0) ccw
  circle A180 centre (0, 0) radius 16.3753
  arc A181 (4.5316, -14.4316) -> (4.7006, -14.1381) centre (4.4567, -14.1931) ccw
  arc A182 (4.665, -13.7348) -> (4.7006, -14.1381) centre (6.1834, -13.8041) ccw
  arc A183 (6.1019, -13.1596) -> (4.665, -13.7348) centre (5.5141, -13.7736) ccw
  arc A184 (6.3545, -13.476) -> (6.1019, -13.1596) centre (5.0508, -14.2576) ccw
  arc A185 (6.3545, -13.476) -> (6.6793, -13.5718) centre (6.5689, -13.3475) ccw
  arc A186 (6.6793, -13.5718) -> (7.1809, -13.3132) centre (0, 0) ccw
  arc A187 (7.1809, -13.3132) -> (7.2913, -12.9931) centre (7.0622, -13.0932) ccw
  arc A188 (7.18, -12.6037) -> (7.2913, -12.9931) centre (8.6841, -12.3845) ccw
  arc A189 (8.4821, -11.767) -> (7.18, -12.6037) centre (8.0211, -12.4811) ccw
  arc A190 (8.79, -12.0299) -> (8.4821, -11.767) centre (7.6578, -13.044) ccw
  arc A191 (8.79, -12.0299) -> (9.1271, -12.0625) centre (8.9762, -11.8631) ccw
  arc A192 (9.1271, -12.0625) -> (9.5706, -11.7136) centre (0, 0) ccw
  arc A193 (1.7185, -15.0284) -> (1.94, -14.7722) centre (1.6901, -14.78) ccw
  arc A194 (1.9814, -14.3695) -> (1.94, -14.7722) centre (3.4592, -14.7249) ccw
  arc A195 (3.5012, -14.0765) -> (1.9814, -14.3695) centre (2.8078, -14.5682) ccw
  arc A196 (3.6893, -14.4351) -> (3.5012, -14.0765) centre (2.2613, -14.9558) ccw
  arc A197 (3.6893, -14.4351) -> (3.9901, -14.5906) centre (3.9242, -14.3494) ccw
  arc A198 (3.9901, -14.5906) -> (4.5316, -14.4316) centre (0, 0) ccw
  dimension "d33" = 32.7507
  measures "d33" diameter of A180
extrude "Extrusion3" add sketch "Skizze3" along normal blind 1 contours A0 A1 A2 A3 A4 A5 A6 A7 A8 A9 A10 A11 A12 A13 A14 A15 A16 A17 A18 A19 A20 A21 A22 A23 A24 A25 A26 A27 A28 A29 A30 A31 A32 A33 A34 A35 A36 A37 A38 A39 A40 A41 A42 A43 A44 A45 A46 A47 A48 A49 A50 A51 A52 A53 A54 A55 A56 A57 A58 A59 A60 A61 A62 A63 A64 A65 A66 A67 A68 A69 A70 A71 A72 A73 A74 A75 A76 A77 A78 A79 A80 A81 A82 A83 A84 A85 A86 A87 A88 A89 A90 A91 A92 A93 A94 A95 A96 A97 A98 A99 A100 A101 A102 A103 A104 A105 A106 A107 A108 A109 A110 A111 A112 A113 A114 A115 A116 A117 A118 A119 A120 A121 A122 A123 A124 A125 A126 A127 A128 A129 A130 A131 A132 A133 A134 A135 A136 A137 A138 A139 A140 A141 A142 A143 A144 A145 A146 A147 A148 A149 A150 A151 A152 A153 A154 A155 A156 A157 A158 A159 A160 A161 A162 A163 A164 A165 A166 A167 A168 A169 A170 A171 A172 A173 A174 A175 A176 A177 A178 A179 A181 A182 A183 A184 A185 A186 A187 A188 A189 A190 A191 A192 A193 A194 A195 A196 A197 A198 | A180 bodies 1
sketch "Skizze17" plane through (0, 8, 0) normal (0, 1, 0) x (-1, 0, 0)
  spline S0 degree 3 poles (13.6382, 4.4313) (13.5302, 4.764) (13.3982, 5.084) (13.1091, 5.6313) (12.979, 5.7983) (12.7664, 6.018) (12.6585, 6.0998) (12.4173, 6.2178) (12.2929, 6.2453) (11.9322, 6.267) (11.6792, 6.209) (10.9713, 5.9696) (10.4381, 5.7266) (9.6899, 5.336) (9.4122, 5.1477) (9.0348, 4.7941) (8.8234, 4.5529) (8.5425, 3.9264) (8.498, 3.6504) (8.4775, 3.1972) (8.4959, 2.9778) (8.559, 2.7826) (8.5803, 2.717) (8.6261, 2.5931) (8.8115, 2.2891) (8.9377, 2.1162) (9.2854, 1.782) (9.4864, 1.6516) (10.0239, 1.4143) (10.3245, 1.381) (10.6864, 1.3735) (11.2116, 1.3812) (12.7231, 1.7144) (12.9818, 1.813) (13.2963, 1.9497) (13.4267, 2.0277) (13.6341, 2.2058) (13.7097, 2.3032) (13.8353, 2.5437) (13.8748, 2.6944) (13.921, 3.1631) (13.8758, 3.4676) (13.7815, 3.9466) (13.7161, 4.1922) (13.6382, 4.4313) knots -0.557189 -0.557189 -0.557189 -0.557189 -0.528825 -0.528825 -0.49746 -0.49746 -0.469449 -0.469449 -0.438886 -0.438886 -0.380684 -0.380684 -0.293014 -0.293014 -0.196609 -0.196609 -0.126355 -0.126355 -0.061556 -0.061556 0 0 0 0.020699 0.020699 0.037386 0.037386 0.056379 0.056379 0.086419 0.086419 0.099545 0.099545 0.108574 0.108574 0.118089 0.118089 0.127425 0.127425 0.139171 0.139171 0.160415 0.160415 0.180805 0.180805 0.180805 0.180805
  spline S1 degree 3 poles (8.4288, 11.6013) (8.146, 11.8071) (7.8511, 11.9884) (7.2955, 12.2611) (7.0921, 12.3198) (6.791, 12.3725) (6.6556, 12.3753) (6.391, 12.329) (6.2743, 12.2782) (5.9697, 12.0837) (5.7991, 11.8881) (5.3671, 11.2782) (5.0786, 10.7683) (4.7028, 10.0125) (4.5889, 9.6969) (4.4914, 9.189) (4.4621, 8.8696) (4.6031, 8.1977) (4.7294, 7.9482) (4.9792, 7.5696) (5.123, 7.4029) (5.2888, 7.2821) (5.3446, 7.2414) (5.4545, 7.1681) (5.7831, 7.0312) (5.9869, 6.9655) (6.4647, 6.8995) (6.7039, 6.9122) (7.2782, 7.0361) (7.5409, 7.1858) (7.8381, 7.3925) (8.2585, 7.7074) (9.2855, 8.8654) (9.4368, 9.0973) (9.6109, 9.3927) (9.6706, 9.5325) (9.7337, 9.7985) (9.7376, 9.9217) (9.6979, 10.1901) (9.6412, 10.3352) (9.4031, 10.7416) (9.1875, 10.9614) (8.8297, 11.2934) (8.6324, 11.4537) (8.4288, 11.6013) knots -0.557189 -0.557189 -0.557189 -0.557189 -0.528825 -0.528825 -0.49746 -0.49746 -0.469449 -0.469449 -0.438886 -0.438886 -0.380684 -0.380684 -0.293014 -0.293014 -0.196609 -0.196609 -0.126355 -0.126355 -0.061556 -0.061556 0 0 0 0.020699 0.020699 0.037386 0.037386 0.056379 0.056379 0.086419 0.086419 0.099545 0.099545 0.108574 0.108574 0.118089 0.118089 0.127425 0.127425 0.139171 0.139171 0.160415 0.160415 0.180805 0.180805 0.180805 0.180805
  spline S2 degree 3 poles (-13.6382, -4.4313) (-13.5302, -4.764) (-13.3982, -5.084) (-13.1091, -5.6313) (-12.979, -5.7983) (-12.7664, -6.018) (-12.6585, -6.0998) (-12.4173, -6.2178) (-12.2929, -6.2453) (-11.9322, -6.267) (-11.6792, -6.209) (-10.9713, -5.9696) (-10.4381, -5.7266) (-9.6899, -5.336) (-9.4122, -5.1477) (-9.0348, -4.7941) (-8.8234, -4.5529) (-8.5425, -3.9264) (-8.498, -3.6504) (-8.4775, -3.1972) (-8.4959, -2.9778) (-8.559, -2.7826) (-8.5803, -2.717) (-8.6261, -2.5931) (-8.8115, -2.2891) (-8.9377, -2.1162) (-9.2854, -1.782) (-9.4864, -1.6516) (-10.0239, -1.4143) (-10.3245, -1.381) (-10.6864, -1.3735) (-11.2116, -1.3812) (-12.7231, -1.7144) (-12.9818, -1.813) (-13.2963, -1.9497) (-13.4267, -2.0277) (-13.6341, -2.2058) (-13.7097, -2.3032) (-13.8353, -2.5437) (-13.8748, -2.6944) (-13.921, -3.1631) (-13.8758, -3.4676) (-13.7815, -3.9466) (-13.7161, -4.1922) (-13.6382, -4.4313) knots -0.557189 -0.557189 -0.557189 -0.557189 -0.528825 -0.528825 -0.49746 -0.49746 -0.469449 -0.469449 -0.438886 -0.438886 -0.380684 -0.380684 -0.293014 -0.293014 -0.196609 -0.196609 -0.126355 -0.126355 -0.061556 -0.061556 0 0 0 0.020699 0.020699 0.037386 0.037386 0.056379 0.056379 0.086419 0.086419 0.099545 0.099545 0.108574 0.108574 0.118089 0.118089 0.127425 0.127425 0.139171 0.139171 0.160415 0.160415 0.180805 0.180805 0.180805 0.180805
  spline S3 degree 3 poles (13.6382, -4.4313) (13.7464, -4.0987) (13.8277, -3.7622) (13.9155, -3.1495) (13.9084, -2.9379) (13.8655, -2.6353) (13.8263, -2.5057) (13.7005, -2.2684) (13.6161, -2.173) (13.337, -1.9434) (13.0982, -1.8416) (12.3848, -1.6193) (11.8106, -1.5025) (10.9757, -1.3786) (10.6404, -1.3678) (10.1272, -1.432) (9.8143, -1.5029) (9.2189, -1.8446) (9.0206, -2.0418) (8.7377, -2.3964) (8.6236, -2.5846) (8.56, -2.7797) (8.5386, -2.8453) (8.5028, -2.9724) (8.4741, -3.3273) (8.4746, -3.5414) (8.5595, -4.0162) (8.6455, -4.2398) (8.9408, -4.7477) (9.1644, -4.9513) (9.4528, -5.1701) (9.8822, -5.4726) (11.3009, -6.0915) (11.5681, -6.1637) (11.9029, -6.238) (12.0543, -6.2516) (12.3268, -6.2294) (12.4451, -6.195) (12.6881, -6.0743) (12.8087, -5.9756) (13.1216, -5.6236) (13.264, -5.3506) (13.4692, -4.9077) (13.5607, -4.6705) (13.6382, -4.4313) knots -0.557189 -0.557189 -0.557189 -0.557189 -0.528825 -0.528825 -0.49746 -0.49746 -0.469449 -0.469449 -0.438886 -0.438886 -0.380684 -0.380684 -0.293014 -0.293014 -0.196609 -0.196609 -0.126355 -0.126355 -0.061556 -0.061556 0 0 0 0.020699 0.020699 0.037386 0.037386 0.056379 0.056379 0.086419 0.086419 0.099545 0.099545 0.108574 0.108574 0.118089 0.118089 0.127425 0.127425 0.139171 0.139171 0.160415 0.160415 0.180805 0.180805 0.180805 0.180805
  spline S4 degree 3 poles (8.4288, -11.6013) (8.7119, -11.3959) (8.9755, -11.1714) (9.4066, -10.7273) (9.5253, -10.552) (9.6685, -10.2819) (9.7129, -10.154) (9.7506, -9.8881) (9.7384, -9.7613) (9.6475, -9.4116) (9.5142, -9.1888) (9.0677, -8.5896) (8.6718, -8.1576) (8.0692, -7.5667) (7.8043, -7.3609) (7.3514, -7.1111) (7.0566, -6.9846) (6.374, -6.9111) (6.0977, -6.954) (5.6604, -7.0746) (5.4575, -7.1598) (5.2913, -7.2802) (5.2354, -7.3207) (5.1318, -7.4026) (4.9, -7.6728) (4.7745, -7.8463) (4.5641, -8.2803) (4.5023, -8.5117) (4.4427, -9.0962) (4.5039, -9.3924) (4.6086, -9.7389) (4.7781, -10.2361) (5.5621, -11.5706) (5.7359, -11.7861) (5.963, -12.043) (6.0775, -12.143) (6.311, -12.2852) (6.427, -12.327) (6.6945, -12.3721) (6.8501, -12.3631) (7.3101, -12.2622) (7.5858, -12.1251) (8.0121, -11.8875) (8.2256, -11.7493) (8.4288, -11.6013) knots -0.557189 -0.557189 -0.557189 -0.557189 -0.528825 -0.528825 -0.49746 -0.49746 -0.469449 -0.469449 -0.438886 -0.438886 -0.380684 -0.380684 -0.293014 -0.293014 -0.196609 -0.196609 -0.126355 -0.126355 -0.061556 -0.061556 0 0 0 0.020699 0.020699 0.037386 0.037386 0.056379 0.056379 0.086419 0.086419 0.099545 0.099545 0.108574 0.108574 0.118089 0.118089 0.127425 0.127425 0.139171 0.139171 0.160415 0.160415 0.180805 0.180805 0.180805 0.180805
  spline S5 degree 3 poles (-8.4288, -11.6013) (-8.146, -11.8071) (-7.8511, -11.9884) (-7.2955, -12.2611) (-7.0921, -12.3198) (-6.791, -12.3725) (-6.6556, -12.3753) (-6.391, -12.329) (-6.2743, -12.2782) (-5.9697, -12.0837) (-5.7991, -11.8881) (-5.3671, -11.2782) (-5.0786, -10.7683) (-4.7028, -10.0125) (-4.5889, -9.6969) (-4.4914, -9.189) (-4.4621, -8.8696) (-4.6031, -8.1977) (-4.7294, -7.9482) (-4.9792, -7.5696) (-5.123, -7.4029) (-5.2888, -7.2821) (-5.3446, -7.2414) (-5.4545, -7.1681) (-5.7831, -7.0312) (-5.9869, -6.9655) (-6.4647, -6.8995) (-6.7039, -6.9122) (-7.2782, -7.0361) (-7.5409, -7.1858) (-7.8381, -7.3925) (-8.2585, -7.7074) (-9.2855, -8.8654) (-9.4368, -9.0973) (-9.6109, -9.3927) (-9.6706, -9.5325) (-9.7337, -9.7985) (-9.7376, -9.9217) (-9.6979, -10.1901) (-9.6412, -10.3352) (-9.4031, -10.7416) (-9.1875, -10.9614) (-8.8297, -11.2934) (-8.6324, -11.4537) (-8.4288, -11.6013) knots -0.557189 -0.557189 -0.557189 -0.557189 -0.528825 -0.528825 -0.49746 -0.49746 -0.469449 -0.469449 -0.438886 -0.438886 -0.380684 -0.380684 -0.293014 -0.293014 -0.196609 -0.196609 -0.126355 -0.126355 -0.061556 -0.061556 0 0 0 0.020699 0.020699 0.037386 0.037386 0.056379 0.056379 0.086419 0.086419 0.099545 0.099545 0.108574 0.108574 0.118089 0.118089 0.127425 0.127425 0.139171 0.139171 0.160415 0.160415 0.180805 0.180805 0.180805 0.180805
  spline S6 degree 3 poles (0, -14.34) (0.3498, -14.3402) (0.6949, -14.3135) (1.3047, -14.2077) (1.5038, -14.1356) (1.7784, -14.0012) (1.8895, -13.9239) (2.0763, -13.7309) (2.141, -13.6212) (2.2731, -13.2848) (2.2961, -13.0262) (2.2871, -12.279) (2.2207, -11.6968) (2.0805, -10.8645) (1.9872, -10.5423) (1.7676, -10.074) (1.6035, -9.7984) (1.0945, -9.3377) (0.8457, -9.2101) (0.421, -9.0506) (0.2067, -9.0002) (0.0015, -9) (-0.0675, -8.9999) (-0.1994, -9.0052) (-0.5458, -9.0876) (-0.7493, -9.1542) (-1.1746, -9.3816) (-1.3607, -9.5325) (-1.7524, -9.9703) (-1.877, -10.2459) (-1.996, -10.5878) (-2.151, -11.0897) (-2.3012, -12.6301) (-2.2873, -12.9067) (-2.2545, -13.248) (-2.2206, -13.3961) (-2.1153, -13.6485) (-2.0461, -13.7504) (-1.8562, -13.9442) (-1.725, -14.0283) (-1.2936, -14.2171) (-0.99, -14.2682) (-0.5053, -14.3266) (-0.2515, -14.3403) (0, -14.34) knots -0.557189 -0.557189 -0.557189 -0.557189 -0.528825 -0.528825 -0.49746 -0.49746 -0.469449 -0.469449 -0.438886 -0.438886 -0.380684 -0.380684 -0.293014 -0.293014 -0.196609 -0.196609 -0.126355 -0.126355 -0.061556 -0.061556 0 0 0 0.020699 0.020699 0.037386 0.037386 0.056379 0.056379 0.086419 0.086419 0.099545 0.099545 0.108574 0.108574 0.118089 0.118089 0.127425 0.127425 0.139171 0.139171 0.160415 0.160415 0.180805 0.180805 0.180805 0.180805
  spline S7 degree 3 poles (-13.6382, 4.4313) (-13.7464, 4.0987) (-13.8277, 3.7622) (-13.9155, 3.1495) (-13.9084, 2.9379) (-13.8655, 2.6353) (-13.8263, 2.5057) (-13.7005, 2.2684) (-13.6161, 2.173) (-13.337, 1.9434) (-13.0982, 1.8416) (-12.3848, 1.6193) (-11.8106, 1.5025) (-10.9757, 1.3786) (-10.6404, 1.3678) (-10.1272, 1.432) (-9.8143, 1.5029) (-9.2189, 1.8446) (-9.0206, 2.0418) (-8.7377, 2.3964) (-8.6236, 2.5846) (-8.56, 2.7797) (-8.5386, 2.8453) (-8.5028, 2.9724) (-8.4741, 3.3273) (-8.4746, 3.5414) (-8.5595, 4.0162) (-8.6455, 4.2398) (-8.9408, 4.7477) (-9.1644, 4.9513) (-9.4528, 5.1701) (-9.8822, 5.4726) (-11.3009, 6.0915) (-11.5681, 6.1637) (-11.9029, 6.238) (-12.0543, 6.2516) (-12.3268, 6.2294) (-12.4451, 6.195) (-12.6881, 6.0743) (-12.8087, 5.9756) (-13.1216, 5.6236) (-13.264, 5.3506) (-13.4692, 4.9077) (-13.5607, 4.6705) (-13.6382, 4.4313) knots -0.557189 -0.557189 -0.557189 -0.557189 -0.528825 -0.528825 -0.49746 -0.49746 -0.469449 -0.469449 -0.438886 -0.438886 -0.380684 -0.380684 -0.293014 -0.293014 -0.196609 -0.196609 -0.126355 -0.126355 -0.061556 -0.061556 0 0 0 0.020699 0.020699 0.037386 0.037386 0.056379 0.056379 0.086419 0.086419 0.099545 0.099545 0.108574 0.108574 0.118089 0.118089 0.127425 0.127425 0.139171 0.139171 0.160415 0.160415 0.180805 0.180805 0.180805 0.180805
  spline S8 degree 3 poles (-8.4288, 11.6013) (-8.7119, 11.3959) (-8.9755, 11.1714) (-9.4066, 10.7273) (-9.5253, 10.552) (-9.6685, 10.2819) (-9.7129, 10.154) (-9.7506, 9.8881) (-9.7384, 9.7613) (-9.6475, 9.4116) (-9.5142, 9.1888) (-9.0677, 8.5896) (-8.6718, 8.1576) (-8.0692, 7.5667) (-7.8043, 7.3609) (-7.3514, 7.1111) (-7.0566, 6.9846) (-6.374, 6.9111) (-6.0977, 6.954) (-5.6604, 7.0746) (-5.4575, 7.1598) (-5.2913, 7.2802) (-5.2354, 7.3207) (-5.1318, 7.4026) (-4.9, 7.6728) (-4.7745, 7.8463) (-4.5641, 8.2803) (-4.5023, 8.5117) (-4.4427, 9.0962) (-4.5039, 9.3924) (-4.6086, 9.7389) (-4.7781, 10.2361) (-5.5621, 11.5706) (-5.7359, 11.7861) (-5.963, 12.043) (-6.0775, 12.143) (-6.311, 12.2852) (-6.427, 12.327) (-6.6945, 12.3721) (-6.8501, 12.3631) (-7.3101, 12.2622) (-7.5858, 12.1251) (-8.0121, 11.8875) (-8.2256, 11.7493) (-8.4288, 11.6013) knots -0.557189 -0.557189 -0.557189 -0.557189 -0.528825 -0.528825 -0.49746 -0.49746 -0.469449 -0.469449 -0.438886 -0.438886 -0.380684 -0.380684 -0.293014 -0.293014 -0.196609 -0.196609 -0.126355 -0.126355 -0.061556 -0.061556 0 0 0 0.020699 0.020699 0.037386 0.037386 0.056379 0.056379 0.086419 0.086419 0.099545 0.099545 0.108574 0.108574 0.118089 0.118089 0.127425 0.127425 0.139171 0.139171 0.160415 0.160415 0.180805 0.180805 0.180805 0.180805
  spline S9 degree 3 poles (0, 14.34) (-0.3498, 14.3402) (-0.6949, 14.3135) (-1.3047, 14.2077) (-1.5038, 14.1356) (-1.7784, 14.0012) (-1.8895, 13.9239) (-2.0763, 13.7309) (-2.141, 13.6212) (-2.2731, 13.2848) (-2.2961, 13.0262) (-2.2871, 12.279) (-2.2207, 11.6968) (-2.0805, 10.8645) (-1.9872, 10.5423) (-1.7676, 10.074) (-1.6035, 9.7984) (-1.0945, 9.3377) (-0.8457, 9.2101) (-0.421, 9.0506) (-0.2067, 9.0002) (-0.0015, 9) (0.0675, 8.9999) (0.1994, 9.0052) (0.5458, 9.0876) (0.7493, 9.1542) (1.1746, 9.3816) (1.3607, 9.5325) (1.7524, 9.9703) (1.877, 10.2459) (1.996, 10.5878) (2.151, 11.0897) (2.3012, 12.6301) (2.2873, 12.9067) (2.2545, 13.248) (2.2206, 13.3961) (2.1153, 13.6485) (2.0461, 13.7504) (1.8562, 13.9442) (1.725, 14.0283) (1.2936, 14.2171) (0.99, 14.2682) (0.5053, 14.3266) (0.2515, 14.3403) (0, 14.34) knots -0.557189 -0.557189 -0.557189 -0.557189 -0.528825 -0.528825 -0.49746 -0.49746 -0.469449 -0.469449 -0.438886 -0.438886 -0.380684 -0.380684 -0.293014 -0.293014 -0.196609 -0.196609 -0.126355 -0.126355 -0.061556 -0.061556 0 0 0 0.020699 0.020699 0.037386 0.037386 0.056379 0.056379 0.086419 0.086419 0.099545 0.099545 0.108574 0.108574 0.118089 0.118089 0.127425 0.127425 0.139171 0.139171 0.160415 0.160415 0.180805 0.180805 0.180805 0.180805
  circle A0 centre (0, 0) radius 16.0986
  circle A1 centre (0, 0) radius 3.6
  line L0 (3.7528, -6.5) -> (7.5056, 0)
  line L1 (7.5056, 0) -> (3.7528, 6.5)
  line L2 (3.7528, 6.5) -> (-3.7528, 6.5)
  line L3 (-3.7528, 6.5) -> (-7.5056, 0)
  line L4 (-7.5056, 0) -> (-3.7528, -6.5)
  line L5 (-3.7528, -6.5) -> (3.7528, -6.5)
  circle A2 centre (0, 0) radius 16.3753
  dimension "d112" = 7.2
  dimension "d113" = 13
  measures "d112" diameter of A1
  measures "d113" distance of L1 L4
extrude "Extrusion18" cut sketch "Skizze17" against normal through all contours A1 bodies 1